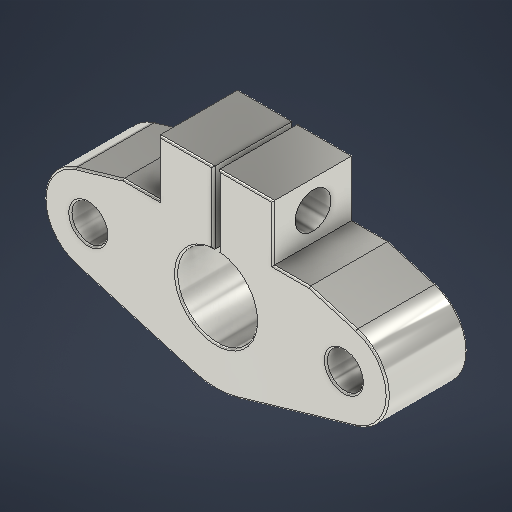
# Autodesk Inventor part: Linear_Shaft_Support_SHF10
Saved by Autodesk Inventor 2025.2 (Build 292293000, 293)
## iProperties
Created: 2025-04-06
Part Number: Linear_Shaft_Support_SHF10
Material: Stainless Steel
Document SubType Name: Modeling
Designer: Tiago
Density: 8 g/cm^3
Appearance: Steel Galvanized
Mass: 32.4649 g
Surface Area: 27.7437 cm^2
Volume: 4.05811 cm^3
Author: Tiago
Autodesk Inventor part; units mm, degrees
ref_plane "YZ Plane" through (0, 0, 0) normal (1, 0, 0) x (0, 1, 0)
ref_plane "XZ Plane" through (0, 0, 0) normal (0, 1, 0) x (-1, 0, 0)
ref_plane "XY Plane" through (0, 0, 0) normal (0, 0, 1) x (1, 0, 0)
sketch "Sketch1" plane through (0, 0, 0) normal (0, 0, 1) x (1, 0, 0)
  circle A0 centre (0, 0) radius 5
  circle A1 centre (0, 0) radius 10
  line L0 (0, -10) -> (0, 14) construction
  line L1 (-16, 0) -> (16, 0) construction
  line L2 (-21.5, 0) -> (21.5, 0) construction
  circle A2 centre (16, 0) radius 2.25
  arc A3 (17.5469, -5.278) -> (17.5469, 5.278) centre (16, 0) ccw
  line L3 (2.8125, -9.5963) -> (17.5469, -5.278)
  circle A4 centre (-16, 0) radius 2.25
  arc A5 (-17.5469, 5.278) -> (-17.5469, -5.278) centre (-16, 0) ccw
  line L4 (-2.8125, -9.5963) -> (-17.5469, -5.278)
  line L5 (0, 14) -> (0, 9.5) construction
  line L6 (0, 9.5) -> (3.1225, 9.5) construction
  line L7 (3.1225, 7) -> (3.1225, 12)
  line L8 (3.1225, 12) -> (3.1225, 14)
  line L9 (3.1225, 14) -> (0, 14) construction
  line L10 (3.1225, 7) -> (7.1414, 7)
  line L11 (7.1414, 7) -> (7.1414, 10.0963)
  line L12 (7.1414, 10.0963) -> (3.1225, 10.0963)
  line L13 (3.1225, 9.5) -> (0.3225, 9.5) construction
  line L14 (0.3225, 9.5) -> (0.3225, 14)
  line L15 (0.3225, 14) -> (3.1225, 14)
  line L16 (3.1225, 14) -> (3.1225, 13)
  line L17 (3.1225, 7) -> (3.1225, 8)
  line L18 (3.1225, 8) -> (3.1225, 10.5)
  line L19 (-6.8775, 10.5) -> (13.1225, 10.5)
  line L20 (3.1225, 13) -> (0.3225, 13)
  line L21 (3.1225, 8) -> (0.3225, 8)
  line L22 (0.3225, 8) -> (0.3225, 9.5)
  line L23 (-3.1225, 7) -> (-3.1225, 12)
  line L24 (-3.1225, 12) -> (-3.1225, 14)
  line L25 (-3.1225, 7) -> (-7.1414, 7)
  line L26 (-7.1414, 7) -> (-7.1414, 10.0963)
  line L27 (-7.1414, 10.0963) -> (-3.1225, 10.0963)
  line L28 (-3.1225, 9.5) -> (-0.3225, 9.5) construction
  line L29 (-0.3225, 9.5) -> (-0.3225, 14)
  line L30 (-0.3225, 14) -> (-3.1225, 14)
  line L31 (-3.1225, 14) -> (-3.1225, 13)
  line L32 (-3.1225, 8) -> (-3.1225, 10.5)
  line L33 (-3.1225, 13) -> (-0.3225, 13)
  line L34 (-3.1225, 8) -> (-0.3225, 8)
  line L35 (-0.3225, 8) -> (-0.3225, 9.5)
  line L36 (3.1225, 7) -> (0.3225, 7)
  line L37 (0.3225, 7) -> (0.3225, 8)
  line L38 (-3.1225, 7) -> (-0.3225, 7)
  line L39 (-0.3225, 7) -> (-0.3225, 8)
  line L40 (-0.3225, 7) -> (-0.3225, 4.9896)
  line L41 (0.3225, 7) -> (0.3225, 4.9896)
  line L42 (7.1414, 7) -> (11.6713, 7)
  line L43 (-7.1414, 7) -> (-11.6713, 7)
  line L44 (-2.8125, 9.5963) -> (-3.1225, 9.5055)
  line L45 (-11.6713, 7) -> (-17.5469, 5.278)
  line L46 (2.8125, 9.5963) -> (3.1225, 9.5055)
  line L47 (11.6713, 7) -> (17.5469, 5.278)
  line L48 (7.1414, 10.0963) -> (7.1414, 14)
  line L49 (3.1225, 14) -> (7.1414, 14)
  line L50 (-3.1225, 14) -> (-7.1414, 14)
  line L51 (-7.1414, 14) -> (-7.1414, 10.0963)
  point P0 (-0.3225, 9.9948)
  point P1 (0.3225, 9.9948)
  point P2 (3.1225, 9.5)
  point P3 (-3.1225, 9.5)
  dimension "di" = 10
  dimension "G" = 20
  dimension "FF" = 24
  dimension "B" = 32
  dimension "WW" = 43
  dimension "d5" = 4.5
  dimension "d6" = 4.5
  dimension "d7" = 5
  dimension "espaço" = 2.8
  dimension "d9" = 1
  dimension "d10" = 1
  dimension "d11" = 2.5
  dimension "d12" = 20
  constraints: 104 end point, 22 symmetric about line, 18 point on line, 11 perpendicular, 11 point on circle, 6 centre point, 6 midpoint, 6 vertical, 5 coincident, 4 horizontal, 4 tangent, 1 collinear, 1 parallel, 2 other
  measures "di" diameter of A0
  measures "G" diameter of A1
  measures "FF" distance of L0.start L0.end
  measures "B" distance of L1.start L1.end
  measures "WW" distance of L2.start L2.end
  measures "d5" diameter of A2
  measures "d6" distance of L0.end L5.end
  measures "d7" distance of L7.start L7.end
  measures "espaço" distance of L6.end L13.end
  measures "d9" distance of L8.end L16.end
  measures "d10" distance of L7.start L17.end
  measures "d11" distance of L17.end L18.end
  measures "d12" distance of L19.start L19.end
extrude "Extrusion1" add sketch "Sketch1" along normal blind 10 contours A0 L41 L36 L10 A1 L25 L38 L40 | L37 L21 L7 L36 | L38 L23 L34 L39 | L7 A1 L10 | L22 L14 A1 L7 L21 | L25 A1 L23 | L34 L23 A1 L29 L35
extrude "Extrusion2" add sketch "Sketch1" along normal blind 10 contours L7 A1 L10 | L42 L47 A3 L3 A1 | A1 L4 A5 L45 L43
extrude "Extrusion3" add sketch "Sketch1" along normal up to surface (10 mm away) contours A1 L7 L12 L11 | L26 L27 L23 A1 | A1 L46 L7 | L12 L7 L19 L48 | L14 L19 L7 L46 A1 | L23 L44 A1 | L51 L50 L24 L23 L27 | A1 L44 L23 L19 L29 | L19 L7 L8 L49 L48 | L14 L20 L8 L7 L19 | L19 L23 L24 L33 L29 | L14 L15 L8 L20 | L30 L29 L33 L24
sketch "Sketch2" plane through (0, 0, 0) normal (1, 0, 0) x (0, 1, 0)
  line L0 (14, 0) -> (4.9896, 0) projected
  line L1 (14, 0) -> (10.5, 0)
  line L2 (10.5, 0) -> (8, 0)
  line L3 (10.5, 0) -> (13, 0)
  line L4 (10.5, 0) -> (10.5, 5) construction
  line L5 (4.9896, 10) -> (14, 10) projected
  circle A0 centre (10.5, 5) radius 2.25
  point P0 (0, 0)
  dimension "d19" = 3.5
  dimension "d20" = 2.5
  dimension "d21" = 2.5
  dimension "d22" = 5
  dimension "d23" = 4.5
  constraints: 8 end point, 3 point on line, 1 centre point, 1 coincident, 1 perpendicular
  measures "d19" distance of L0.start L1.end
  measures "d20" distance of L1.end L2.end
  measures "d21" distance of L1.end L3.end
  measures "d22" distance of L1.end L4.end
  measures "d23" diameter of A0
extrude "Extrusion4" cut sketch "Sketch2" along normal mid plane 20
fillet "Fillet1" radius 0.2 36 edges at (0, -10, 10) (-7.1414, 10.5, 10) (7.1414, 10.5, 10) (-3.732, 14, 10) (3.732, 14, 10) (-3.732, 14, 0) (-7.1414, 10.5, 0) (3.732, 14, 0) (7.1414, 10.5, 0) (-9.4064, 7, 10) (-21.5, 0, 10) (-10.1797, -7.4372, 10) (-14.6091, 6.139, 10) (-21.5, 0, 0) (-10.1797, -7.4372, 0) (0, -10, 0) (10.1797, -7.4372, 0) (21.5, 0, 0) (14.6091, 6.139, 0) (-14.6091, 6.139, 0) (-9.4064, 7, 0) (21.5, 0, 10) (10.1797, -7.4372, 10) (14.6091, 6.139, 10) (9.4064, 7, 10) (9.4064, 7, 0) (0, -5, 0) (13.75, 0, 0) (-18.25, 0, 0) (0, -5, 10) (-0.3225, 9.4948, 10) (0.3225, 9.4948, 10) (-0.3225, 9.4948, 0) (0.3225, 9.4948, 0) (-18.25, 0, 10) (13.75, 0, 10)
equation "\"d20\" = 0.5 * M5"
equation "\"d21\" = 0.5 * M5"
equation "\"SS\" = 5.5"
equation "\"M5\" = 5"
body "Solid1"
